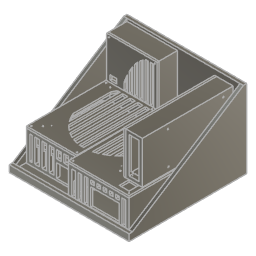
miata-center-console (Autodesk Fusion 360 design; units mm, degrees)
Autodesk Fusion 360 part; units mm, degrees
(part 1 of 2)
sketch "Skizze1" plane through (0, 0, 0) normal (0, 0, 1) x (1, 0, 0) in component "case"
  line L0 (0, 0) -> (178, 0)
  line L1 (178, 0) -> (178, 175)
  line L2 (178, 175) -> (0, 175)
  line L3 (0, 175) -> (0, 0)
  line L4 (5, 170) -> (5, 5)
  line L5 (5, 5) -> (173, 5)
  line L6 (173, 5) -> (173, 170)
  line L7 (173, 170) -> (5, 170)
  line L8 (173, 170) -> (178, 170)
  line L9 (5, 170) -> (0, 170)
  dimension "d1" = 178
  dimension "d2" = 175
  dimension "d3" = -5
  constraint horizontal L0
  constraint vertical L1
  constraint horizontal L2
  constraint vertical L3
  constraint coincident L0.start L3.end
  constraint coincident L1 L8.end
  constraint perpendicular L1 L8
  constraint coincident L3 L9.end
  constraint perpendicular L3 L9
  measures "d1" distance of L0.start L0.end
  measures "d2" distance of L0.start L2.end
extrude "Extrusion1" add sketch "Skizze1" along normal blind 5 makes body 1 in component "case"
extrude "Extrusion2" add sketch "Skizze1" along normal blind 10 contours L0 L1 L3 L4 L5 L6 L8 L9 | L1 L2 L3 L7 L8 L9 bodies 1 in component "case"
extrude "Extrusion3" add sketch "Skizze1" along normal blind 116 contours L1 L2 L3 L7 L8 L9 bodies 1 in component "case"
chamfer "Fase1" distance 165 distance2 106 2 edges at (2.5, 170, 10) (175.5, 170, 10) measured on face at (117, 1.6667, 10) measured on face at (117, 1.6667, 10) on bodies 1 in component "case"
sketch "Skizze2" plane through (0, 0, 5) normal (0, 0, 1) x (-1, 0, 0) in component "light-controller-case"
  line L0 (-173, -170) -> (-5, -170)
  line L1 (-5, -170) -> (-5, -5)
  line L2 (-5, -5) -> (-173, -5)
  line L3 (-173, -5) -> (-173, -170)
  line L4 (-11, -132.7003) -> (-76, -132.7003)
  line L5 (-76, -132.7003) -> (-76, -24.7003)
  line L6 (-76, -24.7003) -> (-11, -24.7003)
  line L7 (-11, -24.7003) -> (-11, -132.7003)
  line L8 (-9, -22.7003) -> (-9, -134.7003)
  line L9 (-9, -134.7003) -> (-78, -134.7003)
  line L10 (-78, -134.7003) -> (-78, -22.7003)
  line L11 (-78, -22.7003) -> (-9, -22.7003)
  line L12 (-6, -19.7003) -> (-6, -137.7003)
  line L13 (-6, -137.7003) -> (-81, -137.7003)
  line L14 (-81, -137.7003) -> (-81, -19.7003)
  line L15 (-81, -19.7003) -> (-6, -19.7003)
  line L16 (-5, -5) -> (-5, -170)
  line L17 (-16, -29.7003) -> (-16, -127.7003) construction
  line L18 (-16, -127.7003) -> (-71, -127.7003) construction
  line L19 (-71, -127.7003) -> (-71, -29.7003) construction
  line L20 (-71, -29.7003) -> (-16, -29.7003) construction
  circle A0 centre (-16, -127.7003) radius 1
  circle A1 centre (-71, -127.7003) radius 1
  circle A2 centre (-16, -29.7003) radius 1
  circle A3 centre (-71, -29.7003) radius 1
  dimension "d41" = 65
  dimension "d42" = 108
  dimension "d43" = -2
  dimension "d44" = -5
  dimension "d45" = 1
  dimension "d52" = 5
  dimension "d54" = 2
  dimension "d55" = 2
  dimension "d56" = 2
  dimension "d57" = 2
  constraint horizontal L4
  constraint vertical L5
  constraint horizontal L6
  constraint vertical L7
  constraint coincident L17.end L18.start
  constraint coincident L18.end L19.start
  constraint coincident L17.start L20.end
  constraint coincident L19.end L20.start
  measures "d41" distance of L4.start L4.end
  measures "d42" distance of L4.start L6.end
  measures "d45" distance of L12.start L16
  measures "d54" diameter of A0
  measures "d55" diameter of A1
  measures "d56" diameter of A2
  measures "d57" diameter of A3
extrude "Extrusion4" add sketch "Skizze2" along normal blind 3 separate body contours L4 L5 L6 L7 | A0 | A1 | A2 | A3 makes body 2 in component "light-controller-case"
extrude "Extrusion5" add sketch "Skizze2" along normal blind 25 contours L8 L9 L10 L11 bodies 2 in component "light-controller-case"
extrude "Extrusion6" add sketch "Skizze2" along normal blind 45 contours L12 L13 L14 L15 bodies 2 in component "light-controller-case"
chamfer "Fase1'" distance 6 angle 45 4 edges at (9, 134.7003, 40) (78, 134.7003, 40) (78, 22.7003, 40) (9, 22.7003, 40) on bodies 2 in component "light-controller-case"
extrude "Extrusion6'" cut sketch "Skizze2" along normal blind 15 from surface at -10 contours A0 | A1 | A2 | A3 bodies 1 in component "case"
extrude "Extrusion7" cut sketch "Skizze2" along normal blind 15 from surface at -10 contours A0 | A1 | A2 | A3 bodies 2 in component "light-controller-case"
sketch "Skizze3" plane through (0, 0, 30) normal (0, 0, 1) x (-1, 0, 0) in component "light-controller-case"
  line L0 (-74, -24.7003) -> (-13, -24.7003)
  line L1 (-11, -26.7003) -> (-11, -130.7003)
  line L2 (-13, -132.7003) -> (-74, -132.7003)
  line L3 (-76, -130.7003) -> (-76, -26.7003)
  line L4 (-78, -28.7003) -> (-78, -128.7003)
  line L5 (-72, -134.7003) -> (-15, -134.7003)
  line L6 (-9, -128.7003) -> (-9, -28.7003)
  line L7 (-15, -22.7003) -> (-72, -22.7003)
  line L8 (-78, -128.7003) -> (-78, -28.7003)
  line L9 (-15, -134.7003) -> (-72, -134.7003)
  line L10 (-9, -28.7003) -> (-9, -128.7003)
  line L11 (-72, -22.7003) -> (-15, -22.7003)
  line L12 (-9.6, -134.1003) -> (-9.6, -23.3003)
  line L13 (-9.6, -23.3003) -> (-77.4, -23.3003)
  line L14 (-77.4, -23.3003) -> (-77.4, -134.1003)
  line L15 (-77.4, -134.1003) -> (-9.6, -134.1003)
  line L16 (-9.6, -47.1003) -> (-77.4, -46.7916)
  line L17 (-9.6, -47.1003) -> (-76, -26.7003) construction
  line L18 (-68.9973, -45.0088) -> (-16.6027, -45.0088)
  line L19 (-16.6027, -45.0088) -> (-16.6027, -28.7918)
  line L20 (-16.6027, -28.7918) -> (-68.9973, -28.7918)
  line L21 (-68.9973, -28.7918) -> (-68.9973, -45.0088)
  line L22 (-68.9973, -45.0088) -> (-16.6027, -28.7918) construction
  line L23 (-16.6027, -45.0088) -> (-68.9973, -28.7918) construction
  line L24 (-74, -132.7003) -> (-72, -134.7003)
  line L25 (-15, -134.7003) -> (-13, -132.7003)
  line L26 (-9, -28.7003) -> (-11, -26.7003)
  line L27 (-11, -130.7003) -> (-9, -128.7003)
  line L28 (-76, -26.7003) -> (-78, -28.7003)
  line L29 (-78, -128.7003) -> (-76, -130.7003)
  line L30 (-13, -24.7003) -> (-15, -22.7003)
  line L31 (-72, -22.7003) -> (-74, -24.7003)
  line L32 (-78, -128.7003) -> (-72, -134.7003)
  line L33 (-15, -134.7003) -> (-9, -128.7003)
  line L34 (-72, -22.7003) -> (-78, -28.7003)
  line L35 (-9, -28.7003) -> (-15, -22.7003)
  line L36 (-77.4364, -128.1367) -> (-71.4364, -134.1367)
  line L37 (-15.5636, -134.1367) -> (-9.5636, -128.1367)
  line L38 (-9.5636, -29.2639) -> (-15.5636, -23.2639)
  line L39 (-71.4364, -23.2639) -> (-77.4364, -29.2639)
  point P0 (-42.8, -36.9003)
  dimension "d67" = 87
  dimension "d262" = -0.797
  dimension "d263" = -0.797
  dimension "d264" = -0.797
  dimension "d265" = -0.797
  constraint coincident L12 L16.start
  constraint coincident L14 L16.end
  constraint coincident L3.end L17.end
  constraint horizontal L18
  constraint perpendicular L18 L19
  constraint parallel L18 L20
  constraint parallel L19 L21
  constraint coincident L22 P0
  constraint coincident L23 P0
  constraint midpoint L17 P0
  measures "d67" distance of L12.start L16.start
extrude "Extrusion8" add sketch "Skizze3" along normal blind 3 separate body contours L0 L13 L38 L39 | L0 L1 L3 L16 L38 L39 | L3 L14 L16 L39 | L1 L12 L16 L38 | L1 L2 L3 L16 L36 L37 | L3 L14 L16 L36 | L1 L12 L16 L37 | L2 L15 L36 L37 makes body 3 in component "light-controller-case"
sketch "Skizze4" plane through (0, 0, 50) normal (0, 0, 1) x (-1, 0, 0) in component "light-controller-case"
  line L0 (-78, -128.7003) -> (-78, -28.7003)
  line L1 (-72, -22.7003) -> (-15, -22.7003)
  line L2 (-9, -28.7003) -> (-9, -128.7003)
  line L3 (-15, -134.7003) -> (-72, -134.7003)
  line L4 (-81, -19.7003) -> (-81, -137.7003)
  line L5 (-81, -137.7003) -> (-6, -137.7003)
  line L6 (-6, -137.7003) -> (-6, -19.7003)
  line L7 (-6, -19.7003) -> (-81, -19.7003)
  line L8 (-81, -19.7003) -> (-81, -137.7003)
  line L9 (-6, -19.7003) -> (-81, -19.7003)
  line L10 (-6, -137.7003) -> (-6, -19.7003)
  line L11 (-81, -137.7003) -> (-6, -137.7003)
  line L12 (-9.5, -23.2003) -> (-77.5, -23.2003) construction
  line L13 (-77.5, -23.2003) -> (-77.5, -134.2003) construction
  line L14 (-77.5, -134.2003) -> (-9.5, -134.2003) construction
  line L15 (-9.5, -134.2003) -> (-9.5, -23.2003) construction
  circle A0 centre (-9.5, -23.2003) radius 1
  circle A1 centre (-77.5, -23.2003) radius 1
  circle A2 centre (-77.5, -134.2003) radius 1
  circle A3 centre (-9.5, -134.2003) radius 1
  line L16 (-78, -28.7003) -> (-72, -22.7003)
  line L17 (-15, -22.7003) -> (-9, -28.7003)
  line L18 (-9, -128.7003) -> (-15, -134.7003)
  line L19 (-72, -134.7003) -> (-78, -128.7003)
  dimension "d68" = -3.5
  dimension "d69" = 2
  dimension "d70" = 2
  dimension "d71" = 2
  dimension "d72" = 2
  constraint coincident L12.start L15.end
  constraint coincident L12.end L13.start
  constraint coincident L13.end L14.start
  constraint coincident L14.end L15.start
  measures "d69" diameter of A0
  measures "d70" diameter of A1
  measures "d71" diameter of A2
  measures "d72" diameter of A3
extrude "Extrusion9" add sketch "Skizze4" along normal blind 3 separate body contours L0 L1 L2 L3 L16 L17 L18 L19 | L4 L5 L6 L7 L8 L9 L10 L11 makes body 4 in component "light-controller-case"
extrude "Extrusion10" cut sketch "Skizze4" against normal blind 5 contours A0 | A1 | A2 | A3 bodies 2 in component "light-controller-case"
sketch "Skizze5" plane through (0, 0, 8) normal (0, 0, 1) x (-1, 0, 0) in component "light-controller-case"
  circle A0 centre (-71, -29.7003) radius 1
  circle A1 centre (-71, -127.7003) radius 1
  circle A2 centre (-16, -29.7003) radius 1
  circle A3 centre (-16, -127.7003) radius 1
  line L0 (-13, -24.7003) -> (-74, -24.7003)
  line L1 (-76, -26.7003) -> (-76, -130.7003)
  line L2 (-74, -132.7003) -> (-13, -132.7003)
  line L3 (-11, -130.7003) -> (-11, -26.7003)
  line L4 (-43.5, -132.7003) -> (-43.5, -24.7003) construction
  line L5 (-65.75, -108.9648) -> (-21.25, -108.9648) construction
  line L6 (-21.25, -108.9648) -> (-21.25, -128.6648) construction
  line L7 (-21.25, -128.6648) -> (-65.75, -128.6648) construction
  line L8 (-65.75, -128.6648) -> (-65.75, -108.9648) construction
  line L9 (-65.75, -108.9648) -> (-21.25, -128.6648) construction
  line L10 (-21.25, -108.9648) -> (-65.75, -128.6648) construction
  line L11 (-68.55, -105.9148) -> (-18.45, -105.9148) construction
  line L12 (-18.45, -105.9148) -> (-18.45, -131.7148) construction
  line L13 (-18.45, -131.7148) -> (-68.55, -131.7148) construction
  line L14 (-68.55, -131.7148) -> (-68.55, -105.9148) construction
  line L15 (-68.55, -105.9148) -> (-18.45, -131.7148) construction
  line L16 (-18.45, -105.9148) -> (-68.55, -131.7148) construction
  circle A4 centre (-21.25, -128.6648) radius 1
  circle A5 centre (-65.75, -128.6648) radius 1
  circle A6 centre (-65.75, -108.9648) radius 1
  circle A7 centre (-21.25, -108.9648) radius 1
  line L17 (-68.55, -79.2481) -> (-18.45, -79.2481) construction
  line L18 (-68.55, -105.0481) -> (-68.55, -79.2481) construction
  line L19 (-18.45, -105.0481) -> (-68.55, -105.0481) construction
  line L20 (-18.45, -79.2481) -> (-18.45, -105.0481) construction
  circle A8 centre (-21.25, -101.9981) radius 1
  circle A9 centre (-21.25, -82.2981) radius 1
  circle A10 centre (-65.75, -82.2981) radius 1
  circle A11 centre (-65.75, -101.9981) radius 1
  line L21 (-68.55, -52.5815) -> (-18.45, -52.5815) construction
  line L22 (-68.55, -78.3815) -> (-68.55, -52.5815) construction
  line L23 (-18.45, -78.3815) -> (-68.55, -78.3815) construction
  line L24 (-18.45, -52.5815) -> (-18.45, -78.3815) construction
  circle A12 centre (-21.25, -75.3315) radius 1
  circle A13 centre (-21.25, -55.6315) radius 1
  circle A14 centre (-65.75, -55.6315) radius 1
  circle A15 centre (-65.75, -75.3315) radius 1
  line L25 (-68.55, -25.9148) -> (-18.45, -25.9148) construction
  line L26 (-68.55, -51.7148) -> (-68.55, -25.9148) construction
  line L27 (-18.45, -51.7148) -> (-68.55, -51.7148) construction
  line L28 (-18.45, -25.9148) -> (-18.45, -51.7148) construction
  circle A16 centre (-21.25, -48.6648) radius 1
  circle A17 centre (-21.25, -28.9648) radius 1
  circle A18 centre (-65.75, -28.9648) radius 1
  circle A19 centre (-65.75, -48.6648) radius 1
  line L29 (-11, -26.7003) -> (-13, -24.7003)
  line L30 (-74, -24.7003) -> (-76, -26.7003)
  line L31 (-76, -130.7003) -> (-74, -132.7003)
  line L32 (-13, -132.7003) -> (-11, -130.7003)
  point P0 (-43.5, -118.8148)
  point P1 (-43.5, -118.8148)
  dimension "d77" = 44.5
  dimension "d78" = 19.7
  dimension "d79" = 50.1
  dimension "d80" = 25.8
  dimension "d81" = 2
  dimension "d82" = 2
  dimension "d83" = 2
  dimension "d84" = 2
  dimension "d87" = 0
  dimension "d88" = 80
  constraint midpoint L2 L4.start
  constraint midpoint L0 L4.end
  constraint horizontal L5
  constraint perpendicular L5 L6
  constraint parallel L5 L7
  constraint parallel L6 L8
  constraint coincident L9 P1
  constraint coincident L10 P1
  constraint coincident L4 P1
  constraint horizontal L11
  constraint perpendicular L11 L12
  constraint parallel L11 L13
  constraint parallel L12 L14
  constraint coincident L15 P1
  constraint coincident L16 P1
  constraint coincident P1 P0
  constraint coincident L6.end L7.start
  constraint coincident L7.end L8.start
  constraint coincident L5.start L8.end
  constraint coincident L5.end L6.start
  measures "d77" distance of L6.end L7.end
  measures "d78" distance of L5.end L6.end
  measures "d79" distance of L12.end L13.end
  measures "d80" distance of L11.end L12.end
  measures "d81" diameter of A4
  measures "d82" diameter of A5
  measures "d83" diameter of A6
  measures "d84" diameter of A7
extrude "Extrusion11" cut sketch "Skizze5" against normal blind 16 contours A4 | A5 | A6 | A7 | A8 | A9 | A10 | A11 | A12 | A13 | A14 | A15 | A16 | A17 | A18 | A19 bodies 2 in component "light-controller-case"
sketch "Skizze6" plane through (0, 0, 33) normal (0, 0, 1) x (-1, 0, 0) in component "light-controller-case"
  line L0 (-68.9973, -45.0088) -> (-68.9973, -28.7918)
  line L1 (-68.9973, -28.7918) -> (-16.6027, -28.7918)
  line L2 (-16.6027, -28.7918) -> (-16.6027, -45.0088)
  line L3 (-16.6027, -45.0088) -> (-68.9973, -45.0088)
  line L4 (-71.4729, -134.1003) -> (-15.5271, -134.1003)
  line L5 (-9.6, -128.1732) -> (-9.6, -29.2274)
  line L6 (-15.5271, -23.3003) -> (-71.4729, -23.3003)
  line L7 (-77.4, -29.2274) -> (-77.4, -128.1732)
  line L8 (-16.1995, -127.4149) -> (-69.6995, -127.4149) construction
  line L9 (-69.6995, -127.4149) -> (-69.6995, -59.1449) construction
  line L10 (-69.6995, -59.1449) -> (-16.1995, -59.1449) construction
  line L11 (-16.1995, -59.1449) -> (-16.1995, -127.4149) construction
  line L12 (-18.5995, -59.1449) -> (-18.5995, -125.0149) construction
  line L13 (-18.5995, -125.0149) -> (-67.2995, -125.0149) construction
  line L14 (-67.2995, -125.0149) -> (-67.2995, -59.1449) construction
  circle A0 centre (-67.2995, -72.4249) radius 1
  circle A1 centre (-18.5995, -74.5449) radius 1
  circle A2 centre (-62.1995, -125.0149) radius 1
  circle A3 centre (-34.3995, -125.0149) radius 1
  line L15 (-15, -134.7003) -> (-9, -128.7003)
  line L16 (-78, -128.7003) -> (-72, -134.7003)
  line L17 (-72, -22.7003) -> (-78, -28.7003)
  line L18 (-9, -28.7003) -> (-15, -22.7003)
  line L19 (-71.4365, -23.2638) -> (-77.4365, -29.2638)
  line L20 (-9.5636, -29.2639) -> (-15.5636, -23.2639)
  line L21 (-15.5636, -134.1367) -> (-9.5636, -128.1367)
  line L22 (-77.4364, -128.1367) -> (-71.4364, -134.1367)
  line L23 (-71.4729, -23.3003) -> (-77.4, -29.2274)
  line L24 (-77.4, -128.1732) -> (-71.4729, -134.1003)
  line L25 (-15.5271, -134.1003) -> (-9.6, -128.1732)
  line L26 (-9.6, -29.2274) -> (-15.5271, -23.3003)
  dimension "d91" = 53.5
  dimension "d92" = 68.27
  dimension "d93" = 2.4
  dimension "d94" = 2
  dimension "d95" = 2
  dimension "d96" = 2
  dimension "d97" = 2
  dimension "d98" = 13.28
  dimension "d99" = 15.4
  dimension "d100" = 7.5
  dimension "d101" = 18.2
  dimension "d258" = -0.797
  dimension "d259" = -0.797
  dimension "d260" = -0.797
  dimension "d261" = -0.797
  constraint horizontal L8
  constraint vertical L9
  constraint horizontal L10
  constraint vertical L11
  constraint coincident L14 A0.centre
  constraint coincident L12 A1.centre
  constraint coincident L13 A2.centre
  constraint coincident L13 A3.centre
  measures "d91" distance of L8.start L8.end
  measures "d92" distance of L8.start L10.end
  measures "d94" diameter of A0
  measures "d95" diameter of A1
  measures "d96" diameter of A2
  measures "d97" diameter of A3
  measures "d98" distance of L14.end A0.centre
  measures "d99" distance of L12.start A1.centre
  measures "d100" distance of L9 A2.centre
  measures "d101" distance of L11 A3.centre
extrude "Extrusion12" cut sketch "Skizze6" against normal blind 5 contours A0 | A1 | A2 | A3 bodies 3 in component "light-controller-case"
sketch "Skizze1 (2)" plane through (0, 0, 5) normal (0, 0, 1) x (-1, 0, 0) in component "computer-case"
  circle A0 centre (-71, -29.7003) radius 1
  circle A1 centre (-71, -127.7003) radius 1
  circle A2 centre (-16, -29.7003) radius 1
  circle A3 centre (-16, -127.7003) radius 1
  line L0 (-5, -170) -> (-5, -5)
  line L1 (-5, -5) -> (-173, -5)
  line L2 (-173, -5) -> (-173, -170)
  line L3 (-173, -170) -> (-5, -170)
  line L4 (-82, -169) -> (-172, -169)
  line L5 (-172, -169) -> (-172, -6)
  line L6 (-172, -6) -> (-82, -6)
  line L7 (-82, -6) -> (-82, -169)
  line L8 (-173, -170) -> (-173, -5)
  line L9 (-81, -19.7003) -> (-81, -137.7003)
  line L10 (-162, -16) -> (-92, -16) construction
  line L11 (-92, -16) -> (-92, -159) construction
  line L12 (-92, -159) -> (-162, -159) construction
  line L13 (-162, -159) -> (-162, -16) construction
  circle A4 centre (-92, -159) radius 1
  circle A5 centre (-162, -159) radius 1
  circle A6 centre (-92, -16) radius 1
  circle A7 centre (-162, -16) radius 1
  line L14 (-5, -170) -> (-173, -170)
  line L15 (-85, -166) -> (-169, -166)
  line L16 (-169, -166) -> (-169, -9)
  line L17 (-169, -9) -> (-85, -9)
  line L18 (-85, -9) -> (-85, -166)
  dimension "d104" = 90
  dimension "d106" = 1
  dimension "d107" = 10
  dimension "d108" = 2
  dimension "d109" = 2
  dimension "d110" = 2
  dimension "d111" = 2
  dimension "d114" = 1
  dimension "d116" = 1
  dimension "d117" = 3
  constraint horizontal L4
  constraint vertical L5
  constraint horizontal L6
  constraint vertical L7
  constraint coincident L11.end L12.start
  constraint coincident L12.end L13.start
  constraint coincident L10.end L11.start
  constraint coincident L10.start L13.end
  measures "d104" distance of L4.start L4.end
  measures "d106" distance of L5 L8
  measures "d108" diameter of A4
  measures "d109" diameter of A5
  measures "d110" diameter of A6
  measures "d111" diameter of A7
  measures "d114" distance of L4 L14
  measures "d116" distance of L1 L6
extrude "Extrusion1'" add sketch "Skizze1 (2)" along normal blind 3 separate body contours L4 L5 L6 L7 | L15 L16 L17 L18 makes body 5 in component "computer-case"
extrude "Extrusion7'" cut sketch "Skizze1 (2)" against normal blind 10 contours A4 | A5 | A6 | A7 bodies 1 in component "case"
extrude "Extrusion2'" add sketch "Skizze1 (2)" along normal blind 45 contours L4 L5 L6 L7 bodies 5 in component "computer-case"
chamfer "Fase1''" distance 6 angle 45 4 edges at (85, 9, 29) (85, 166, 29) (169, 166, 29) (169, 9, 29) on bodies 5 in component "computer-case"
sketch "Skizze2 (2)" plane through (0, 0, 50) normal (0, 0, 1) x (-1, 0, 0) in component "computer-case"
  line L0 (-163, -9) -> (-91, -9)
  line L1 (-85, -15) -> (-85, -160)
  line L2 (-91, -166) -> (-163, -166)
  line L3 (-169, -160) -> (-169, -15)
  line L4 (-82, -6) -> (-172, -6)
  line L5 (-172, -6) -> (-172, -169)
  line L6 (-172, -169) -> (-82, -169)
  line L7 (-82, -169) -> (-82, -6)
  line L8 (-172, -6) -> (-172, -169)
  line L9 (-172, -169) -> (-82, -169)
  line L10 (-82, -169) -> (-82, -6)
  line L11 (-82, -6) -> (-172, -6)
  line L12 (-168.5, -165.5) -> (-85.5, -165.5) construction
  line L13 (-85.5, -165.5) -> (-85.5, -9.5) construction
  line L14 (-85.5, -9.5) -> (-168.5, -9.5) construction
  line L15 (-168.5, -9.5) -> (-168.5, -165.5) construction
  circle A0 centre (-168.5, -9.5) radius 1
  circle A1 centre (-85.5, -9.5) radius 1
  circle A2 centre (-85.5, -165.5) radius 1
  circle A3 centre (-168.5, -165.5) radius 1
  line L16 (-91, -9) -> (-85, -15)
  line L17 (-85, -160) -> (-91, -166)
  line L18 (-163, -166) -> (-169, -160)
  line L19 (-169, -15) -> (-163, -9)
  dimension "d120" = -3.5
  dimension "d121" = 2
  dimension "d122" = 2
  dimension "d123" = 2
  dimension "d124" = 2
  constraint coincident L14.end L15.start
  constraint coincident L13.end L14.start
  constraint coincident L12.end L13.start
  constraint coincident L12.start L15.end
  measures "d121" diameter of A0
  measures "d122" diameter of A1
  measures "d123" diameter of A2
  measures "d124" diameter of A3
extrude "Extrusion3'" add sketch "Skizze2 (2)" along normal blind 3 separate body contours L0 L1 L2 L3 L16 L17 L18 L19 | L4 L5 L6 L7 L8 L9 L10 L11 makes body 6 in component "computer-case"
extrude "Extrusion4'" cut sketch "Skizze2 (2)" against normal blind 7 contours A0 | A1 | A2 | A3 bodies 5 in component "computer-case"
sketch "Skizze4 (2)" plane through (0, 0, 8) normal (0, 0, 1) x (-1, 0, 0) in component "computer-case"
  line L0 (-169, -15) -> (-169, -160)
  line L1 (-163, -166) -> (-91, -166)
  line L2 (-85, -160) -> (-85, -15)
  line L3 (-91, -9) -> (-163, -9)
  circle A0 centre (-162, -16) radius 1
  circle A1 centre (-162, -159) radius 1
  circle A2 centre (-92, -16) radius 1
  circle A3 centre (-92, -159) radius 1
  line L4 (-85, -15) -> (-169, -160) construction
  line L5 (-160.95, -33.275) -> (-93.05, -33.275) construction
  line L6 (-93.05, -33.275) -> (-93.05, -141.725) construction
  line L7 (-93.05, -141.725) -> (-160.95, -141.725) construction
  line L8 (-160.95, -141.725) -> (-160.95, -33.275) construction
  line L9 (-160.95, -33.275) -> (-93.05, -141.725) construction
  line L10 (-93.05, -33.275) -> (-160.95, -141.725) construction
  circle A4 centre (-93.05, -141.725) radius 1
  circle A5 centre (-160.95, -141.725) radius 1
  circle A6 centre (-93.05, -33.275) radius 1
  circle A7 centre (-160.95, -33.275) radius 1
  line L11 (-163, -9) -> (-169, -15)
  line L12 (-169, -160) -> (-163, -166)
  line L13 (-91, -166) -> (-85, -160)
  line L14 (-85, -15) -> (-91, -9)
  point P0 (-127, -87.5)
  dimension "d131" = 108.45
  dimension "d132" = 67.9
  dimension "d133" = 2
  dimension "d134" = 2
  dimension "d135" = 2
  dimension "d136" = 2
  constraint coincident L2.end L4.start
  constraint coincident L0.end L4.end
  constraint horizontal L5
  constraint perpendicular L5 L6
  constraint parallel L5 L7
  constraint parallel L6 L8
  constraint coincident L9 P0
  constraint coincident L10 P0
  constraint midpoint L4 P0
  constraint coincident L6.end L7.start
  constraint coincident L7.end L8.start
  constraint coincident L5.end L6.start
  constraint coincident L5.start L8.end
  measures "d131" distance of L5.start L7.end
  measures "d132" distance of L6.end L7.end
  measures "d133" diameter of A4
  measures "d134" diameter of A5
  measures "d135" diameter of A6
  measures "d136" diameter of A7
extrude "Extrusion5'" cut sketch "Skizze4 (2)" against normal blind 7 contours A4 | A5 | A6 | A7 bodies 5 in component "computer-case"
sketch "Skizze1 (3)" plane through (0, 0, 5) normal (0, 0, 1) x (-1, 0, 0) in component "power-supply"
  circle A0 centre (-71, -29.7003) radius 1
  circle A1 centre (-71, -127.7003) radius 1
  circle A2 centre (-16, -29.7003) radius 1
  circle A3 centre (-16, -127.7003) radius 1
  line L0 (-5, -170) -> (-5, -5)
  line L1 (-5, -5) -> (-173, -5)
  line L2 (-173, -5) -> (-173, -170)
  line L3 (-173, -170) -> (-5, -170)
  circle A4 centre (-162, -16) radius 1
  circle A5 centre (-92, -159) radius 1
  circle A6 centre (-92, -16) radius 1
  circle A7 centre (-162, -159) radius 1
  line L4 (-81, -137.7003) -> (-6, -137.7003)
  line L5 (-82, -6) -> (-82, -169)
  line L6 (-6, -169) -> (-81, -169)
  line L7 (-81, -169) -> (-81, -138.7003)
  line L8 (-81, -138.7003) -> (-6, -138.7003)
  line L9 (-6, -138.7003) -> (-6, -169)
  line L10 (-82, -169) -> (-82, -6)
  line L11 (-5, -5) -> (-5, -170)
  line L12 (-5, -170) -> (-173, -170)
  line L13 (-73, -146.7003) -> (-14, -146.7003) construction
  line L14 (-14, -146.7003) -> (-14, -161) construction
  line L15 (-14, -161) -> (-73, -161) construction
  line L16 (-73, -161) -> (-73, -146.7003) construction
  circle A8 centre (-14, -161) radius 1
  circle A9 centre (-14, -146.7003) radius 1
  circle A10 centre (-73, -146.7003) radius 1
  circle A11 centre (-73, -161) radius 1
  line L17 (-78, -141.7003) -> (-9, -141.7003)
  line L18 (-9, -141.7003) -> (-9, -166)
  line L19 (-9, -166) -> (-78, -166)
  line L20 (-78, -166) -> (-78, -141.7003)
  line L21 (-9, -141.7003) -> (-6, -141.7003)
  line L22 (-78, -141.7003) -> (-81, -141.7003)
  circle A12 centre (-14, -146.7003) radius 2.6
  circle A13 centre (-73, -146.7003) radius 2.6
  circle A14 centre (-73, -161) radius 2.6
  circle A15 centre (-14, -161) radius 2.6
  dimension "d141" = 1
  dimension "d142" = 1
  dimension "d143" = 1
  dimension "d144" = 1
  dimension "d145" = 8
  dimension "d146" = 2
  dimension "d147" = 2
  dimension "d148" = 2
  dimension "d149" = 2
  dimension "d150" = 3
  dimension "d274" = 5.2
  dimension "d275" = 5.2
  dimension "d276" = 5.2
  dimension "d277" = 5.2
  constraint horizontal L6
  constraint vertical L7
  constraint horizontal L8
  constraint vertical L9
  constraint coincident L14.end L15.start
  constraint coincident L13.end L14.start
  constraint coincident L13.start L16.end
  constraint coincident L15.end L16.start
  constraint coincident L9 L21.end
  constraint perpendicular L9 L21
  constraint coincident L7 L22.end
  constraint perpendicular L7 L22
  constraint concentric A9 A12
  constraint concentric A10 A13
  constraint concentric A11 A14
  constraint concentric A8 A15
  measures "d141" distance of L7 L10
  measures "d142" distance of L9 L11
  measures "d143" distance of L6 L12
  measures "d144" distance of L4 L8
  measures "d146" diameter of A8
  measures "d147" diameter of A9
  measures "d148" diameter of A10
  measures "d149" diameter of A11
  measures "d274" diameter of A12
  measures "d275" diameter of A13
  measures "d276" diameter of A14
  measures "d277" diameter of A15
extrude "Extrusion1''" add sketch "Skizze1 (3)" along normal blind 3 separate body contours L17 L18 L19 L20 | A8 | A9 | A10 | A11 | A12 | A13 | A14 | A15 makes body 7 in component "power-supply"
extrude "Extrusion2''" add sketch "Skizze1 (3)" along normal blind 105 contours L6 L7 L9 L18 L19 L20 L21 L22 bodies 7 in component "power-supply"
sketch "Skizze2 (3)" plane through (0, 166, 0) normal (0, -1, 0) x (1, 0, 0) in component "power-supply"
  line L0 (9, 8) -> (78, 8)
  line L1 (78, 8) -> (78, 110)
  line L2 (78, 110) -> (9, 110)
  line L3 (9, 110) -> (9, 8)
  line L4 (43.5, 8) -> (43.5, 110) construction
  line L5 (65.1, 45.997) -> (21.9, 45.997) construction
  line L6 (21.9, 45.997) -> (21.9, 67.217) construction
  line L7 (21.9, 67.217) -> (65.1, 67.217) construction
  line L8 (65.1, 67.217) -> (65.1, 45.997) construction
  line L9 (65.1, 45.997) -> (21.9, 67.217) construction
  line L10 (21.9, 45.997) -> (65.1, 67.217) construction
  line L11 (9, 43) -> (78, 43) construction
  line L12 (70.25, 75.4473) -> (16.75, 75.4473) construction
  line L13 (16.75, 75.4473) -> (16.75, 104.1473) construction
  line L14 (16.75, 104.1473) -> (70.25, 104.1473) construction
  line L15 (70.25, 104.1473) -> (70.25, 75.4473) construction
  line L16 (70.25, 75.4473) -> (16.75, 104.1473) construction
  line L17 (16.75, 75.4473) -> (70.25, 104.1473) construction
  line L18 (25.75, 104.1473) -> (25.75, 75.4473) construction
  line L19 (60.05, 104.1473) -> (60.05, 75.4473) construction
  line L20 (25.75, 78.2073) -> (60.05, 78.2073) construction
  line L21 (25.75, 96.7873) -> (60.05, 96.7873) construction
  circle A0 centre (25.75, 96.7873) radius 1
  circle A1 centre (60.05, 96.7873) radius 1
  circle A2 centre (25.75, 78.2073) radius 1
  circle A3 centre (60.05, 78.2073) radius 1
  line L22 (28.48, 67.217) -> (28.48, 45.997) construction
  line L23 (58.52, 67.217) -> (58.52, 45.997) construction
  line L24 (28.48, 48.547) -> (58.52, 48.547) construction
  line L25 (28.48, 64.667) -> (58.52, 64.667) construction
  circle A4 centre (28.48, 48.547) radius 1
  circle A5 centre (58.52, 48.547) radius 1
  circle A6 centre (58.52, 64.667) radius 1
  circle A7 centre (28.48, 64.667) radius 1
  line L26 (71, 11.9281) -> (16, 11.9281)
  line L27 (16, 11.9281) -> (16, 36.9281)
  line L28 (16, 36.9281) -> (71, 36.9281)
  line L29 (71, 36.9281) -> (71, 11.9281)
  line L30 (71, 11.9281) -> (16, 36.9281) construction
  line L31 (16, 11.9281) -> (71, 36.9281) construction
  point P0 (43.5, 56.607)
  point P1 (78, 8)
  point P2 (43.5, 89.7973)
  point P3 (43.5, 24.4281)
  dimension "d155" = 43.2
  dimension "d156" = 21.22
  dimension "d157" = 35
  dimension "d158" = 53.5
  dimension "d159" = 28.7
  dimension "d160" = 9
  dimension "d161" = 10.2
  dimension "d162" = 7.36
  dimension "d163" = 2.76
  dimension "d164" = 2
  dimension "d165" = 2
  dimension "d166" = 2
  dimension "d167" = 2
  dimension "d168" = 6.58
  dimension "d169" = 6.58
  dimension "d170" = 2.55
  dimension "d171" = 2.55
  dimension "d172" = 2
  dimension "d173" = 2
  dimension "d174" = 2
  dimension "d175" = 2
  dimension "d327" = 55
  dimension "d328" = 25
  constraint midpoint L0 L4.start
  constraint midpoint L2 L4.end
  constraint horizontal L5
  constraint perpendicular L5 L6
  constraint parallel L5 L7
  constraint parallel L6 L8
  constraint coincident L9 P0
  constraint coincident L10 P0
  constraint coincident L4 P0
  constraint coincident L3 L11.start
  constraint coincident L1 L11.end
  constraint perpendicular L1 L11
  constraint horizontal L12
  constraint perpendicular L12 L13
  constraint parallel L12 L14
  constraint parallel L13 L15
  constraint coincident L16 P2
  constraint coincident L17 P2
  constraint coincident L4 P2
  constraint coincident L14 L18.start
  constraint coincident L12 L18.end
  constraint perpendicular L12 L18
  constraint coincident L14 L19.start
  constraint coincident L12 L19.end
  constraint perpendicular L12 L19
  constraint coincident L18 L20.start
  constraint coincident L19 L20.end
  constraint perpendicular L19 L20
  constraint coincident L18 L21.start
  constraint coincident L19 L21.end
  constraint perpendicular L19 L21
  constraint coincident L21.start A0.centre
  constraint coincident L21.end A1.centre
  constraint coincident L20.start A2.centre
  constraint coincident L20.end A3.centre
  constraint coincident L7 L22.start
  constraint coincident L5 L22.end
  constraint perpendicular L5 L22
  constraint coincident L7 L23.start
  constraint coincident L5 L23.end
  constraint perpendicular L5 L23
  constraint coincident L22 L24.start
  constraint coincident L23 L24.end
  constraint perpendicular L23 L24
  constraint coincident L22 L25.start
  constraint coincident L23 L25.end
  constraint perpendicular L23 L25
  constraint coincident L24.start A4.centre
  constraint coincident L24.end A5.centre
  constraint coincident L25.end A6.centre
  constraint coincident L25.start A7.centre
  constraint horizontal L26
  constraint perpendicular L26 L27
  constraint parallel L26 L28
  constraint parallel L27 L29
  constraint coincident L30 P3
  constraint coincident L31 P3
  constraint coincident L4 P3
  measures "d155" distance of L6.end L7.end
  measures "d156" distance of L5.end L6.end
  measures "d157" distance of L11.end P1
  measures "d158" distance of L13.end L14.end
  measures "d159" distance of L12.end L13.end
  measures "d160" distance of L13 L18
  measures "d161" distance of L15 L19
  measures "d162" distance of L14 L21
  measures "d163" distance of L12 L20
  measures "d164" diameter of A0
  measures "d165" diameter of A1
  measures "d166" diameter of A2
  measures "d167" diameter of A3
  measures "d168" distance of L5.end L22.end
  measures "d169" distance of L5.start L23.end
  measures "d170" distance of L23.start L25.end
  measures "d171" distance of L23.end L24.end
  measures "d172" diameter of A4
  measures "d173" diameter of A5
  measures "d174" diameter of A6
  measures "d175" diameter of A7
  measures "d327" distance of L27.end L28.end
  measures "d328" distance of L26.end L27.end
extrude "Extrusion3''" cut sketch "Skizze2 (3)" against normal blind 5 contours A0 | A1 | A2 | A3 | A4 | A5 | A6 | A7 bodies 7 in component "power-supply"
extrude "Extrusion4''" add sketch "Skizze1 (3)" along normal blind 108 separate body contours L7 L8 L9 L17 L21 L22 makes body 8 in component "power-supply"
extrude "Extrusion6''" add sketch "Skizze1 (3)" along normal blind 3 from surface at 105 contours L6 L7 L9 L18 L19 L20 L21 L22 | L17 L18 L19 L20 | A8 | A9 | A10 | A11 | A12 | A13 | A14 | A15 bodies 7 in component "power-supply"
chamfer "Fase1'''" distance 6 angle 45 4 edges at (9, 153.8501, 110) (78, 153.8501, 110) (9, 153.8501, 8) (78, 153.8501, 8) on bodies 7 in component "power-supply"
sketch "Skizze3 (2)" plane through (0, 138.7003, 0) normal (0, -1, 0) x (1, 0, 0) in component "power-supply"
  line L0 (6, 5) -> (81, 5)
  line L1 (81, 5) -> (81, 113)
  line L2 (81, 113) -> (6, 113)
  line L3 (6, 113) -> (6, 5)
  line L4 (9.5, 8.5) -> (77.5, 8.5) construction
  line L5 (77.5, 8.5) -> (77.5, 109.5) construction
  line L6 (77.5, 109.5) -> (9.5, 109.5) construction
  line L7 (9.5, 109.5) -> (9.5, 8.5) construction
  circle A0 centre (77.5, 109.5) radius 1
  circle A1 centre (9.5, 109.5) radius 1
  circle A2 centre (77.5, 8.5) radius 1
  circle A3 centre (9.5, 8.5) radius 1
  dimension "d180" = -3.5
  dimension "d181" = 2
  dimension "d182" = 2
  dimension "d183" = 2
  dimension "d184" = 2
  constraint coincident L5.end L6.start
  constraint coincident L6.end L7.start
  constraint coincident L4.end L5.start
  constraint coincident L4.start L7.end
  measures "d181" diameter of A0
  measures "d182" diameter of A1
  measures "d183" diameter of A2
  measures "d184" diameter of A3
extrude "Extrusion5''" cut sketch "Skizze3 (2)" against normal blind 10 contours A0 | A1 | A2 | A3 bodies 7 8 in component "power-supply"
sketch "Skizze1 (4)" plane through (0, 0, 53) normal (0, 0, 1) x (-1, 0, 0) in component "fan-holder"
  circle A0 centre (-77.5, -134.2003) radius 1
  circle A1 centre (-9.5, -134.2003) radius 1
  circle A2 centre (-9.5, -23.2003) radius 1
  circle A3 centre (-77.5, -23.2003) radius 1
  line L0 (-81, -137.7003) -> (-6, -137.7003)
  line L1 (-6, -137.7003) -> (-6, -19.7003)
  line L2 (-6, -19.7003) -> (-81, -19.7003)
  line L3 (-81, -19.7003) -> (-81, -137.7003)
  circle A4 centre (-168.5, -165.5) radius 1
  circle A5 centre (-168.5, -9.5) radius 1
  circle A6 centre (-85.5, -165.5) radius 1
  circle A7 centre (-85.5, -9.5) radius 1
  line L4 (-82, -6) -> (-172, -6)
  line L5 (-172, -6) -> (-172, -169)
  line L6 (-172, -169) -> (-82, -169)
  line L7 (-82, -169) -> (-82, -6)
  line L8 (-6, -94.9771) -> (-172, -94.9771) construction
  line L9 (-138.419, -162.9077) -> (-13.419, -162.9077)
  line L10 (-13.419, -162.9077) -> (-13.419, -26.793)
  line L11 (-13.419, -26.793) -> (-138.419, -26.793)
  line L12 (-138.419, -26.793) -> (-138.419, -162.9077)
  line L13 (-138.419, -162.9077) -> (-13.419, -26.793) construction
  line L14 (-13.419, -162.9077) -> (-138.419, -26.793) construction
  line L15 (-81, -137.7003) -> (-82, -137.7003)
  point P0 (-75.919, -94.8504)
  dimension "d190" = 125
  constraint coincident L1 L8.start
  constraint coincident L5 L8.end
  constraint perpendicular L5 L8
  constraint horizontal L9
  constraint perpendicular L9 L10
  constraint parallel L9 L11
  constraint parallel L10 L12
  constraint coincident L13 P0
  constraint coincident L14 P0
  constraint coincident L0.start L3.end
  constraint coincident L7 L15.end
  constraint perpendicular L7 L15
  measures "d190" distance of L10.end L11.end
extrude "Extrusion1'''" add sketch "Skizze1 (4)" along normal blind 60 separate body contours A0 | L0 L3 L10 L11 | L3 L7 L11 L15 | L7 L9 L11 L12 makes body 9 in component "fan-holder"
chamfer "Fase1''''" distance 110 distance2 55 1 edges at (75.919, 26.793, 113) measured on face at (35.946, 63.7621, 113) on bodies 9 in component "fan-holder"
sketch "Skizze2 (4)" plane through (0, -17.8414, 35.6828) normal (0, -0.447214, 0.894427) x (1, 0, 0) in component "fan-holder"
  line L0 (138.419, 49.9028) -> (138.419, 172.8865)
  line L1 (138.419, 172.8865) -> (13.419, 172.8865)
  line L2 (13.419, 172.8865) -> (13.419, 49.9028)
  line L3 (13.419, 49.9028) -> (138.419, 49.9028)
  line L4 (13.419, 49.9028) -> (138.419, 172.8865) construction
  line L5 (127.919, 59.3947) -> (23.919, 59.3947) construction
  line L6 (23.919, 59.3947) -> (23.919, 163.3947) construction
  line L7 (23.919, 163.3947) -> (127.919, 163.3947) construction
  line L8 (127.919, 163.3947) -> (127.919, 59.3947) construction
  line L9 (127.919, 59.3947) -> (23.919, 163.3947) construction
  line L10 (23.919, 59.3947) -> (127.919, 163.3947) construction
  circle A0 centre (75.919, 111.3947) radius 57
  circle A1 centre (127.919, 163.3947) radius 1
  circle A2 centre (23.919, 163.3947) radius 1
  circle A3 centre (23.919, 59.3947) radius 1
  circle A4 centre (127.919, 59.3947) radius 1
  point P0 (75.919, 111.3947)
  dimension "d195" = 104
  dimension "d196" = 104
  dimension "d197" = 114
  dimension "d305" = 2
  dimension "d306" = 2
  dimension "d307" = 2
  dimension "d308" = 2
  constraint coincident L2.end L3.start
  constraint coincident L0.end L1.start
  constraint horizontal L5
  constraint perpendicular L5 L6
  constraint parallel L5 L7
  constraint parallel L6 L8
  constraint coincident L9 P0
  constraint coincident L10 P0
  constraint midpoint L4 P0
  constraint coincident P0 A0.centre
  constraint coincident L7.end L8.start
  constraint coincident L6.end L7.start
  constraint coincident L5.end L6.start
  constraint coincident L5.start L8.end
  measures "d195" distance of L6.end L7.end
  measures "d196" distance of L5.end L6.end
  measures "d197" diameter of A0
  measures "d305" diameter of A1
  measures "d306" diameter of A2
  measures "d307" diameter of A3
  measures "d308" diameter of A4
extrude "Extrusion17" cut sketch "Skizze2 (4)" against normal blind 10 contours A1 | A2 | A3 | A4 bodies 4 in component "light-controller-case"
extrude "Extrusion10'" cut sketch "Skizze2 (4)" against normal blind 10 contours A1 | A2 | A3 | A4 bodies 6 in component "computer-case"
extrude "Extrusion3'''" cut sketch "Skizze2 (4)" against normal blind 10 contours A1 | A2 | A3 | A4 bodies 9 in component "fan-holder"
extrude "Extrusion2'''" cut sketch "Skizze2 (4)" against normal blind 80 contours A0 bodies 9 in component "fan-holder"
fillet "Abrundung1" radius 2.5 tangency weight 1.44037 1 edges at (53.9259, 137.7003, 91.2717) on bodies 9 in component "fan-holder"
sketch "Skizze1 (5)" plane through (0, 0, 53) normal (0, 0, 1) x (-1, 0, 0) in component "cutouts"
  circle A0 centre (-168.5, -165.5) radius 1
  circle A1 centre (-168.5, -9.5) radius 1
  circle A2 centre (-85.5, -165.5) radius 1
  circle A3 centre (-85.5, -9.5) radius 1
  line L0 (-82, -6) -> (-172, -6)
  line L1 (-172, -6) -> (-172, -169)
  line L2 (-172, -169) -> (-82, -169)
  line L3 (-82, -169) -> (-82, -6)
  ellipse E0 centre (-75.919, -98.043) end of major axis (-75.919, -34.3151) minor radius 57 (-28.8224, -133.9407) -> (-82, -161.4072) ccw
  line L4 (-88.0723, -169) -> (-88.0723, -6)
  line L5 (-139.7953, -165.3651) -> (-143.7953, -165.3651)
  line L6 (-143.7953, -165.3651) -> (-143.7953, -27.1982)
  line L7 (-143.7953, -27.1982) -> (-139.7953, -27.1982)
  line L8 (-139.7953, -27.1982) -> (-139.7953, -165.3651)
  line L9 (-128.5453, -165.3651) -> (-132.5453, -165.3651)
  line L10 (-128.5453, -27.1982) -> (-128.5453, -165.3651)
  line L11 (-132.5453, -165.3651) -> (-132.5453, -27.1982)
  line L12 (-117.2953, -165.3651) -> (-121.2953, -165.3651)
  line L13 (-117.2953, -27.1982) -> (-117.2953, -165.3651)
  line L14 (-121.2953, -165.3651) -> (-121.2953, -27.1982)
  line L15 (-106.0453, -165.3651) -> (-110.0453, -165.3651)
  line L16 (-106.0453, -27.1982) -> (-106.0453, -165.3651)
  line L17 (-110.0453, -165.3651) -> (-110.0453, -27.1982)
  ellipse E1 centre (-127.919, -39.9052) end of major axis (-127.919, -38.7872) minor radius 1 (-127.1786, -39.1537) -> (-128.6593, -39.1537) ccw
  line L18 (-127.1786, -39.1537) -> (-128.6593, -39.1537)
  line L19 (-94.7953, -165.3651) -> (-98.7953, -165.3651)
  line L20 (-94.7953, -27.1982) -> (-94.7953, -165.3651)
  line L21 (-98.7953, -165.3651) -> (-98.7953, -27.1982)
  dimension "d204" = -6.0723
  dimension "d205" = 4
  dimension "d208" = 45
  dimension "d209" = 0
  constraint horizontal L5
  constraint vertical L6
  constraint horizontal L7
  constraint vertical L8
  measures "d205" distance of L5.start L5.end
extrude "Extrusion6'''" cut sketch "Skizze1 (5)" against normal blind 10 contours E0 L4 L20 | E0 L16 L21 | E0 L13 L17 | E0 L10 L14 | E0 L11 bodies 6 in component "computer-case"
sketch "Skizze2 (5)" plane through (0, 0, 53) normal (0, 0, 1) x (-1, 0, 0) in component "cutouts"
  circle A0 centre (-77.5, -134.2003) radius 1
  circle A1 centre (-9.5, -134.2003) radius 1
  circle A2 centre (-9.5, -23.2003) radius 1
  circle A3 centre (-77.5, -23.2003) radius 1
  line L0 (-81, -137.7003) -> (-6, -137.7003)
  line L1 (-6, -137.7003) -> (-6, -19.7003)
  line L2 (-6, -19.7003) -> (-81, -19.7003)
  line L3 (-81, -19.7003) -> (-81, -137.7003)
  ellipse E0 centre (-75.919, -98.043) end of major axis (-75.919, -34.3151) minor radius 57 (-28.8224, -133.9407) -> (-82, -161.4072) ccw
  line L4 (-76, -19.7003) -> (-76, -132.7003)
  line L5 (-76, -132.7003) -> (-6, -132.7003)
  line L6 (-20.6845, -132.7003) -> (-24.6845, -132.7003)
  line L7 (-24.6845, -132.7003) -> (-24.6845, -26.862)
  line L8 (-24.6845, -26.862) -> (-20.6845, -26.862)
  line L9 (-20.6845, -26.862) -> (-20.6845, -132.7003)
  line L10 (-35.9345, -132.7003) -> (-35.9345, -26.862)
  line L11 (-31.9345, -26.862) -> (-31.9345, -132.7003)
  line L12 (-47.1845, -132.7003) -> (-47.1845, -26.862)
  line L13 (-43.1845, -26.862) -> (-43.1845, -132.7003)
  line L14 (-58.4345, -132.7003) -> (-58.4345, -26.862)
  line L15 (-54.4345, -26.862) -> (-54.4345, -132.7003)
  ellipse E1 centre (-23.919, -39.9052) end of major axis (-23.919, -38.7872) minor radius 1 (-23.1786, -39.1537) -> (-24.6593, -39.1537) ccw
  line L16 (-23.1786, -39.1537) -> (-24.6593, -39.1537)
  line L17 (-69.6845, -132.7003) -> (-69.6845, -26.862)
  line L18 (-65.6845, -26.862) -> (-65.6845, -132.7003)
  dimension "d212" = -5
  dimension "d213" = 4
  dimension "d216" = -45
  dimension "d217" = 0
  constraint horizontal L6
  constraint vertical L7
  constraint horizontal L8
  constraint vertical L9
  constraint coincident L5 L6.start
  measures "d213" distance of L6.start L6.end
extrude "Extrusion13" cut sketch "Skizze2 (5)" against normal blind 10 contours E0 L4 L5 L17 | E0 L5 L14 L18 | E0 L5 L7 L11 | E0 L5 L12 L15 | E0 L5 L10 L13 bodies 4 in component "light-controller-case"
sketch "Skizze3 (3)" plane through (0, 138.7003, 0) normal (0, -1, 0) x (1, 0, 0) in component "cutouts"
  circle A0 centre (9.5, 109.5) radius 1
  circle A1 centre (9.5, 8.5) radius 1
  circle A2 centre (77.5, 109.5) radius 1
  circle A3 centre (77.5, 8.5) radius 1
  line L0 (6, 5) -> (81, 5)
  line L1 (81, 5) -> (81, 113)
  line L2 (81, 113) -> (6, 113)
  line L3 (6, 113) -> (6, 5)
  spline S0 degree 3 poles (82, 109.8605) (80.6061, 110.2067) (79.1904, 110.437) (75.5462, 110.7112) (73.2859, 110.573) (70.1332, 109.9501) (69.2069, 109.7128) (65.0201, 108.4054) (61.9533, 106.7745) (57.9048, 103.8871) (56.7256, 102.9409) (52.6184, 99.3125) (49.9581, 96.3109) (47.553, 93.117) (45.3874, 90.2412) (43.4266, 87.2048) (39.771, 80.8325) (38.0887, 77.492) (33.4659, 67.2715) (30.9435, 60.2012) (28.8224, 53) knots 0.219289 0.219289 0.219289 0.219289 0.666314 0.666314 1.366916 1.366916 1.66351 1.66351 2.733019 2.733019 3.199117 3.199117 4.42386 4.42386 4.42386 5.526632 5.526632 6.665095 6.665095 8.94058 8.94058 8.94058 8.94058
  line L4 (76, 5) -> (76, 108)
  line L5 (76, 108) -> (6, 108)
  line L6 (28.8224, 53) -> (81, 53)
  line L7 (28.9027, 108) -> (31.9027, 108)
  line L8 (31.9027, 108) -> (31.9027, 40.6431)
  line L9 (31.9027, 40.6431) -> (28.9027, 40.6431)
  line L10 (28.9027, 40.6431) -> (28.9027, 108)
  line L11 (39.7027, 108) -> (39.7027, 40.6431)
  line L12 (36.7027, 40.6431) -> (36.7027, 108)
  line L13 (47.5027, 108) -> (47.5027, 40.6431)
  line L14 (44.5027, 40.6431) -> (44.5027, 108)
  line L15 (55.3027, 108) -> (55.3027, 40.6431)
  line L16 (52.3027, 40.6431) -> (52.3027, 108)
  line L17 (63.1027, 108) -> (63.1027, 40.6431)
  line L18 (60.1027, 40.6431) -> (60.1027, 108)
  line L19 (70.9027, 108) -> (70.9027, 40.6431)
  line L20 (67.9027, 40.6431) -> (67.9027, 108)
  dimension "d220" = -5
  dimension "d221" = 3
  dimension "d224" = 39
  dimension "d225" = 0
  constraint coincident S0.end L6.start
  constraint coincident L1 L6.end
  constraint perpendicular L1 L6
  constraint horizontal L7
  constraint vertical L8
  constraint horizontal L9
  constraint vertical L10
  constraint coincident L5 L7.start
  measures "d221" distance of L7.start L7.end
extrude "Extrusion7''" cut sketch "Skizze3 (3)" against normal blind 10 contours L4 L5 L6 L19 | S0 L5 L6 L17 L20 | S0 L6 L8 L12 | S0 L6 L15 L18 | S0 L6 L11 L14 | S0 L6 L13 L16 bodies 8 in component "power-supply"
extrude "Extrusion8'" cut sketch "Skizze1 (3)" along normal blind 15 from surface at -7 contours A8 | A9 | A10 | A11 bodies 1 in component "case"
extrude "Extrusion8''" cut sketch "Skizze1 (3)" along normal blind 15 from surface at -7 contours A8 | A9 | A10 | A11 bodies 7 in component "power-supply"
extrude "Extrusion9'" cut sketch "Skizze1 (3)" along normal blind 8 from surface at 3 contours A12 | A13 | A14 | A15 bodies 7 in component "power-supply"
sketch "Skizze4 (3)" plane through (0, 19.7003, 0) normal (0, -1, 0) x (1, 0, 0) in component "cutouts"
  line L0 (6, 5) -> (81, 5)
  line L1 (81, 5) -> (81, 50)
  line L2 (81, 50) -> (6, 50)
  line L3 (6, 50) -> (6, 5)
  line L4 (11, 10) -> (76, 10)
  line L5 (76, 10) -> (76, 45)
  line L6 (76, 45) -> (11, 45)
  line L7 (11, 45) -> (11, 10)
  line L8 (14.2165, 47.8988) -> (18.2165, 47.8988)
  line L9 (18.2165, 47.8988) -> (18.2165, 8.178)
  line L10 (18.2165, 8.178) -> (14.2165, 8.178)
  line L11 (14.2165, 8.178) -> (14.2165, 47.8988)
  line L12 (29.0165, 47.8988) -> (29.0165, 8.178)
  line L13 (25.0165, 8.178) -> (25.0165, 47.8988)
  line L14 (39.8165, 47.8988) -> (39.8165, 8.178)
  line L15 (35.8165, 8.178) -> (35.8165, 47.8988)
  line L16 (50.6165, 47.8988) -> (50.6165, 8.178)
  line L17 (46.6165, 8.178) -> (46.6165, 47.8988)
  line L18 (61.4165, 47.8988) -> (61.4165, 8.178)
  line L19 (57.4165, 8.178) -> (57.4165, 47.8988)
  line L20 (72.2165, 47.8988) -> (72.2165, 8.178)
  line L21 (68.2165, 8.178) -> (68.2165, 47.8988)
  line L22 (50.6165, 28) -> (76, 28)
  line L23 (76, 10) -> (76, 5)
  line L24 (50.6165, 8.178) -> (50.6165, 5)
  line L25 (50.6165, 8) -> (76, 8)
  line L26 (50.6165, 33) -> (76, 33)
  dimension "d228" = -5
  dimension "d229" = 4
  dimension "d232" = 54
  dimension "d233" = 0
  dimension "d234" = 3
  dimension "d235" = 20
  dimension "d236" = 5
  constraint horizontal L8
  constraint vertical L9
  constraint horizontal L10
  constraint vertical L11
  constraint coincident L16 L22.start
  constraint coincident L5 L22.end
  constraint perpendicular L5 L22
  constraint coincident L0 L23.end
  constraint perpendicular L0 L23
  constraint coincident L0 L24.end
  constraint perpendicular L0 L24
  constraint coincident L24 L25.start
  constraint coincident L23 L25.end
  constraint perpendicular L23 L25
  constraint coincident L16 L26.start
  constraint coincident L5 L26.end
  constraint perpendicular L5 L26
  measures "d229" distance of L8.start L8.end
  measures "d234" distance of L23.end L25.end
  measures "d235" distance of L22.end L25.end
  measures "d236" distance of L22.end L26.end
extrude "Extrusion14" cut sketch "Skizze4 (3)" against normal blind 10 contours L4 L16 L23 L24 L25 | L4 L5 L20 L22 | L4 L16 L19 L22 | L4 L20 L21 L22 | L4 L6 L14 L17 | L4 L18 L19 L22 | L4 L18 L21 L22 | L5 L6 L20 L26 | L6 L16 L19 L26 | L4 L6 L12 L15 | L6 L18 L21 L26 | L4 L6 L9 L13 | L4 L6 L7 L11 bodies 2 in component "light-controller-case"
sketch "Skizze5 (2)" plane through (82, 0, 0) normal (-1, 0, 0) x (0, -1, 0) in component "cutouts"
  line L0 (-169, 5) -> (-6, 5)
  line L1 (-6, 5) -> (-6, 50)
  line L2 (-6, 50) -> (-169, 50)
  line L3 (-169, 50) -> (-169, 5)
  line L4 (-9, 8) -> (-19.5, 8)
  line L5 (-19.5, 8) -> (-19.5, 28)
  line L6 (-19.5, 28) -> (-9, 28)
  line L7 (-9, 28) -> (-9, 8)
  dimension "d239" = 20
  dimension "d240" = 10.5
  dimension "d241" = 3
  dimension "d242" = 3
  constraint horizontal L4
  constraint vertical L5
  constraint horizontal L6
  constraint vertical L7
  measures "d239" distance of L4.start L6.end
  measures "d240" distance of L4.start L4.end
  measures "d241" distance of L1 L4.start
  measures "d242" distance of L0 L4.start
extrude "Extrusion7'''" cut sketch "Skizze5 (2)" against normal blind 10 contours L4 L5 L6 L7 bodies 5 in component "computer-case"